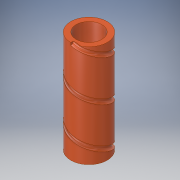
# Autodesk Inventor part: InnerThreadedFocusTube
Saved by Autodesk Inventor 2019.3 (Build 233278000, 278)
## iProperties
Created: 2018-12-30
Part Number: InnerThreadedFocusTube
Material: PBT Plastic
Document SubType Name: Modeling
Designer: steele
Density: 1.31 g/cm^3
Appearance: Smooth - Light Orange
Author: steele
Autodesk Inventor part; units mm, degrees
ref_plane "YZ Plane" through (0, 0, 0) normal (1, 0, 0) x (0, 1, 0)
ref_plane "XZ Plane" through (0, 0, 0) normal (0, 1, 0) x (-1, 0, 0)
ref_plane "XY Plane" through (0, 0, 0) normal (0, 0, 1) x (1, 0, 0)
sketch "Sketch1" plane through (0, 0, 0) normal (0, 1, 0) x (-1, 0, 0)
  circle A0 centre (0, 0) radius 22.606
  circle A1 centre (0, 0) radius 16.002
  dimension "d4" = 32.004
  dimension "d5" = 45.212
  constraints: 2 centre point, 2 coincident
  measures "d4" diameter of A1
  measures "d5" diameter of A0
extrude "Extrusion1" add sketch "Sketch1" against normal blind 127
sketch "Sketch2" plane through (0, 0, 0) normal (1, 0, 0) x (0, 1, 0)
  line L0 (0, 22.606) -> (-127, 22.606) projected
  circle A0 centre (0, 22.606) radius 3.175
  line L1 (0, 22.606) -> (0, -22.606) construction
  point P0 (0, 0)
  dimension "d18" = 6.35
  dimension "d23" = 0
  constraints: 1 centre point, 1 point on line
  measures "d18" diameter of A0
  measures "d23" distance from line of A0.centre L1
coil "Coil1" sketch "Sketch2" operation cut axis through (0, -10, 0) along (0, -1, 0) pitch 50.8 turns 2.5 hand left
sketch "Sketch13" plane through (0, -127, 0) normal (0, -1, 0) x (1, 0, 0)
  circle A0 centre (0, 0) radius 25.146 construction
  arc A1 (8.6509, -20.8852) -> (0, -22.606) centre (0, 0) ccw construction
  line L0 (-1.3947, -15.9411) -> (-2.1121, -25.0571)
  line L1 (1.3947, -15.9411) -> (2.1121, -25.0571)
  line L2 (0, 0) -> (0, -25.146) construction
  circle A2 centre (0, 0) radius 16.002 construction
  arc A3 (-1.3947, -15.9411) -> (1.3947, -15.9411) centre (0, 0) ccw
  arc A4 (-2.1121, -25.0571) -> (2.1121, -25.0571) centre (0, 0) ccw
  dimension "d48" = 2.54
  dimension "d49" = 4.5
  dimension "d50" = 4.5
  constraints: 9 point on circle, 6 end point, 3 centre point, 3 coincident, 1 vertical
  measures "d48" radial gap between concentric circles of A0 A1
  measures "d49" angle of L0 L2
  measures "d50" angle of L1 L2
extrude "Extrusion6" add sketch "Sketch13" against normal blind 50.8
sketch "Sketch10" plane through (0, -127, 0) normal (0, -1, 0) x (1, 0, 0)
  line L0 (0, 0) -> (0, -22.606) construction
  arc A0 (8.6509, -20.8852) -> (0, -22.606) centre (0, 0) ccw construction
  arc A1 (0, -15.875) -> (3.175, -15.5543) centre (0, 0) ccw
  line L1 (3.175, -15.5543) -> (3.175, -25.781)
  line L2 (3.175, -25.781) -> (0, -25.781)
  arc A2 (-3.175, -15.5543) -> (0, -15.875) centre (0, 0) ccw
  line L3 (-3.175, -15.5543) -> (-3.175, -25.781)
  line L4 (-3.175, -25.781) -> (0, -25.781)
  dimension "d37" = 3.175
  dimension "d38" = 31.75
  dimension "d40" = 3.175
  constraints: 10 end point, 5 point on circle, 2 centre point, 2 symmetric about line, 1 coincident, 1 horizontal, 1 point on line, 1 vertical, 1 other
  measures "d37" distance between parallel lines of L1 L0
  measures "d38" diameter of A1
  measures "d40" distance from line of L0.end L2
equation "\"d49\" = 0.5 * angleForSlot"
equation "\"d50\" = 0.5 * angleForSlot"
equation "\"angleForSlot\" = 9deg"
body "Solid1"
